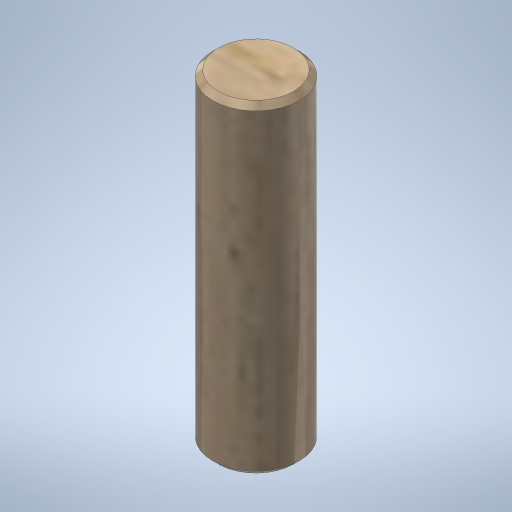
# Autodesk Inventor part: Dowel 30x8
Saved by Autodesk Inventor 2024 (Build 280153000, 153)
## iProperties
RuleStatus: InUse
Created: 2009-08-20
Part Number: Dowel 30x8
Description: Dowel
Document SubType Name: Modeling
Designer: Saulius Dereskeviciu
Density: 0.544 g/cm^3
Material: TMB 01
Appearance: F01
Author: Saulius Dereskeviciu
Autodesk Inventor part; units mm, degrees
ref_plane "YZ Plane" through (0, 0, 0) normal (1, 0, 0) x (0, 1, 0)
ref_plane "XZ Plane" through (0, 0, 0) normal (0, 1, 0) x (-1, 0, 0)
ref_plane "XY Plane" through (0, 0, 0) normal (0, 0, 1) x (1, 0, 0)
sketch "Sketch1" plane through (0, 0, 0) normal (0, 0, 1) x (1, 0, 0)
  circle A0 centre (0, 0) radius 4
  dimension "D" = 8
  constraints: 1 centre point, 1 coincident
  measures "D" diameter of A0
extrude "Extrusion1" add sketch "Sketch1" along normal blind 20 and the other way blind 10
chamfer "Chamfer1" distance 0.5 angle 45 2 edges at (-4, 0, 20) (-4, 0, -10)
sketch "Sketch2" plane through (0, 0, 0) normal (0, 0, 1) x (1, 0, 0)
  circle A0 centre (0, 0) radius 4
  dimension "d8" = 8
  constraints: 1 centre point, 1 coincident
  measures "d8" diameter of A0
extrude "Extrusion2" add sketch "Sketch2" along normal blind 30 and the other way blind 12 separate body
